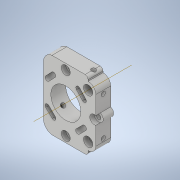
# Autodesk Inventor part: 20_Cube_Insert_Kinematic_VCAmount_Base_Thorlabs_Cage_smaller
Saved by Autodesk Inventor 2022.3 (Build 263350000, 350)
## iProperties
Created: 2019-07-01
Part Number: 20_Cube_Insert_Kinematic_VCAmount_Base_Thorlabs_Cage_smaller
Material: Generic
Document SubType Name: Modeling
Designer: diederichbenedict
Density: 1 g/cm^3
Appearance: Default
Author: diederichbenedict
Autodesk Inventor part; units mm, degrees
ref_plane "YZ Plane" through (0, 0, 0) normal (1, 0, 0) x (0, 1, 0)
ref_plane "Work Plane1" through (0, 0, 10) normal (0, 0, 1) x (1, 0, 0)
sketch "Sketch1" plane through (0, 0, 10) normal (0, 0, 1) x (1, 0, 0)
  line L0 (-4.0299, -0.3538) -> (-2.2322, 1.4439) construction
  arc A0 (-1.4439, 2.2322) -> (-2.2322, 1.4439) centre (-0.9299, 0.9299) ccw construction
  line L1 (-1.4439, 2.2322) -> (0.3538, 4.0299) construction
  line L2 (-37.8299, 42.8299) -> (-37.8299, 37.8299) construction
  line L3 (-37.8299, 37.8299) -> (-42.9208, 37.8299) construction
  line L4 (-37.8299, 42.2137) -> (-37.8299, 45.8299) construction
  line L5 (-37.8299, 45.8299) -> (-4.0299, 45.8299) construction
  line L6 (-4.0299, 45.8299) -> (-4.0299, 42.2137) construction
  line L7 (-4.0299, 4.0299) -> (0.3538, 4.0299) projected
  circle A1 centre (-20.9299, 20.9299) radius 17.5 projected
  line L8 (-20.9299, 58.9723) -> (17.1124, 20.9299) construction
  line L9 (17.1124, 20.9299) -> (-20.9299, -17.1124) construction
  line L10 (-20.9299, -17.1124) -> (-58.9723, 20.9299) construction
  line L11 (-58.9723, 20.9299) -> (-20.9299, 58.9723) construction
  line L12 (-20.9299, 58.9723) -> (-20.9299, -17.1124) construction
  line L13 (17.1124, 20.9299) -> (-58.9723, 20.9299) construction
  line L14 (-20.9299, 58.9723) -> (32.8701, 58.9723) construction
  line L15 (-43.4299, 43.4299) -> (1.5701, 43.4299) construction
  line L16 (1.5701, 43.4299) -> (1.5701, -1.5701) construction
  line L17 (1.5701, -1.5701) -> (-43.4299, -1.5701) construction
  line L18 (-43.4299, -1.5701) -> (-43.4299, 43.4299) construction
  line L19 (-43.4299, 43.4299) -> (1.5701, -1.5701) construction
  line L20 (1.5701, 43.4299) -> (-43.4299, -1.5701) construction
  line L21 (-43.4299, 5.3876) -> (-43.4299, 36.4723)
  line L22 (-43.4299, 36.4723) -> (-36.4723, 43.4299)
  line L23 (-36.4723, 43.4299) -> (-5.3876, 43.4299)
  line L24 (-5.3876, 43.4299) -> (1.5701, 36.4723)
  line L25 (1.5701, 36.4723) -> (1.5701, 5.3876)
  line L26 (1.5701, 5.3876) -> (-5.3876, -1.5701)
  line L27 (-5.3876, -1.5701) -> (-36.4723, -1.5701)
  line L28 (-36.4723, -1.5701) -> (-43.4299, 5.3876)
  line L29 (-4.0299, 42.2137) -> (-37.8299, 42.2137) projected
  line L30 (-4.0299, -0.3538) -> (-4.0299, 4.0299) projected
  point P0 (-37.8299, 4.0299)
  point P1 (-20.9299, 20.9299)
  dimension "d18" = 53.8
  dimension "d19" = 45
  dimension "d20" = 53.8
  dimension "d21" = 45
  dimension "d22" = 45
  constraints: 42 end point, 15 point on line, 5 midpoint, 4 parallel, 3 perpendicular, 2 horizontal, 1 equal length
  measures "d18" distance of L8.start L8.end
  measures "d19" angle of L8 L14
  measures "d20" distance of L8.end L9.end
  measures "d21" distance of L16.end L17.end
  measures "d22" distance of L15.end L16.end
extrude "Extrusion1" add sketch "Sketch1" along normal blind 10 contours L30 L26 L27 L28 L21 L22 L29 L24 L25 L7 | L7 L26 L30 | L29 L22 L23 L24 | A1
ref_plane "Work Plane2" through (-40.9959, 0.8639, 22.2359) normal (0, 0, 1) x (1, 0, 0)
sketch "Sketch3" plane through (0, 0, 10) normal (0, 0, -1) x (-1, 0, 0)
  line L0 (37.8299, -0.4701) -> (37.8299, 4.0299) construction
  line L1 (4.0299, 4.0299) -> (4.0299, -0.4701) construction
  line L2 (37.8299, -0.4701) -> (37.8299, 1.1886) construction
  line L3 (4.0299, -3.9701) -> (4.0299, -0.3538) construction
  line L4 (45.8299, 4.0299) -> (42.2137, 4.0299) construction
  line L5 (-0.3538, 4.0299) -> (-3.9701, 4.0299) construction
  line L6 (-3.9701, 37.8299) -> (-0.3538, 37.8299) construction
  line L7 (4.0299, 42.2137) -> (4.0299, 45.8299) construction
  line L8 (37.8299, 45.8299) -> (37.8299, 42.2137) construction
  line L9 (42.2137, 37.8299) -> (45.8299, 37.8299) construction
  line L10 (40.4657, 37.7299) -> (45.8299, 37.7299)
  line L11 (45.8299, 37.7299) -> (45.8299, 4.1299)
  line L12 (45.8299, 4.1299) -> (40.4657, 4.1299)
  line L13 (40.4657, 4.1299) -> (40.4657, 37.7299)
  line L14 (37.7299, 2.4952) -> (4.1299, 2.4952)
  line L15 (4.1299, 2.4952) -> (4.1299, -3.9701)
  line L16 (4.1299, -3.9701) -> (37.7299, -3.9701)
  line L17 (37.7299, -3.9701) -> (37.7299, 2.4952)
  line L18 (1.8946, 4.1299) -> (-3.9701, 4.1299)
  line L19 (-3.9701, 4.1299) -> (-3.9701, 37.7299)
  line L20 (-3.9701, 37.7299) -> (1.8946, 37.7299)
  line L21 (1.8946, 37.7299) -> (1.8946, 4.1299)
  line L22 (4.1299, 40.7326) -> (37.7299, 40.7326)
  line L23 (37.7299, 40.7326) -> (37.7299, 45.8299)
  line L24 (37.7299, 45.8299) -> (4.1299, 45.8299)
  line L25 (4.1299, 45.8299) -> (4.1299, 40.7326)
  point P0 (0, 0)
  dimension "d23" = 0.1
  dimension "d24" = 0.1
  dimension "d25" = 0.1
  dimension "d26" = 0.1
  dimension "d27" = 0.1
  constraints: 32 end point, 8 parallel, 4 horizontal, 4 perpendicular, 3 point on line
  measures "d23" distance between parallel lines of L8 L23
  measures "d24" distance between parallel lines of L7 L25
  measures "d25" distance between parallel lines of L6 L20
  measures "d26" distance between parallel lines of L5 L18
  measures "d27" distance between parallel lines of L1 L15
extrude "Extrusion3" add sketch "Sketch3" against normal up to surface (10 mm away)
sketch "Sketch4" plane through (0, 0, 20) normal (0, 0, 1) x (1, 0, 0)
  line L0 (3.9701, 4.1299) -> (0.3124, 4.1299) projected
  line L1 (3.9701, 37.7299) -> (3.9701, 4.1299) projected
  line L2 (0.3124, 37.7299) -> (3.9701, 37.7299) projected
  line L3 (0.3124, 37.7299) -> (-4.1299, 42.1723) projected
  line L4 (-4.1299, 45.8299) -> (-4.1299, 42.1723) projected
  line L5 (-37.7299, 45.8299) -> (-4.1299, 45.8299) projected
  line L6 (-37.7299, 42.1723) -> (-37.7299, 45.8299) projected
  line L7 (-37.7299, 42.1723) -> (-42.1723, 37.7299) projected
  line L8 (-45.8299, 37.7299) -> (-42.1723, 37.7299) projected
  line L9 (-45.8299, 4.1299) -> (-45.8299, 37.7299) projected
  line L10 (-42.1723, 4.1299) -> (-45.8299, 4.1299) projected
  line L11 (-42.1723, 4.1299) -> (-37.7299, -0.3124) projected
  line L12 (-37.7299, -3.9701) -> (-37.7299, -0.3124) projected
  line L13 (-4.1299, -3.9701) -> (-37.7299, -3.9701) projected
  line L14 (-4.1299, -0.3124) -> (-4.1299, -3.9701) projected
  line L15 (-4.1299, -0.3124) -> (0.3124, 4.1299) projected
  line L16 (-3.9799, 45.9799) -> (-3.9799, 42.2344)
  line L17 (-3.9799, 42.2344) -> (0.3745, 37.8799)
  line L18 (0.3745, 37.8799) -> (4.1201, 37.8799)
  line L19 (4.1201, 37.8799) -> (4.1201, 3.9799)
  line L20 (4.1201, 3.9799) -> (0.3745, 3.9799)
  line L21 (0.3745, 3.9799) -> (-3.9799, -0.3745)
  line L22 (-3.9799, -0.3745) -> (-3.9799, -4.1201)
  line L23 (-3.9799, -4.1201) -> (-37.8799, -4.1201)
  line L24 (-37.8799, -4.1201) -> (-37.8799, -0.3745)
  line L25 (-37.8799, -0.3745) -> (-42.2344, 3.9799)
  line L26 (-42.2344, 3.9799) -> (-45.9799, 3.9799)
  line L27 (-45.9799, 3.9799) -> (-45.9799, 37.8799)
  line L28 (-45.9799, 37.8799) -> (-42.2344, 37.8799)
  line L29 (-42.2344, 37.8799) -> (-37.8799, 42.2344)
  line L30 (-37.8799, 42.2344) -> (-37.8799, 45.9799)
  line L31 (-37.8799, 45.9799) -> (-3.9799, 45.9799)
  point P0 (0, 0)
  dimension "d34" = 0.15
  constraints: 32 end point, 15 other
  measures "d34" distance between parallel lines of L5 L31
extrude "Extrusion4" add sketch "Sketch4" against normal up to surface (10 mm away)
sketch "Sketch8" plane through (0, 0, 20) normal (0, 0, 1) x (1, 0, 0)
  circle A0 centre (-20.9299, 20.9299) radius 10
  line L0 (4.1201, 37.8799) -> (4.1201, 3.9799) projected
  line L1 (-37.8799, 45.9799) -> (-3.9799, 45.9799) projected
  point P0 (0, 0)
  point P1 (4.1201, 20.9299)
  point P2 (-20.9299, 45.9799)
  dimension "d61" = 20
  constraints: 2 midpoint, 1 centre point, 1 horizontal alignment, 1 vertical alignment
  measures "d61" diameter of A0
ref_plane "Work Plane3" through (-40.0572, 1.8027, 20) normal (-0.7071068, 0.7071068, 0) x (0.7071068, 0.7071068, 0)
sketch "Sketch5" plane through (0, 0, 20) normal (0, 0, 1) x (1, 0, 0)
  circle A0 centre (-20.9299, 20.9299) radius 29.7458 construction
  line L0 (4.1201, 37.8799) -> (4.1201, 3.9799) projected
  line L1 (-37.8799, 45.9799) -> (-3.9799, 45.9799) projected
  line L2 (-34.9299, 6.9299) -> (-6.9299, 6.9299) construction
  line L3 (-6.9299, 6.9299) -> (-6.9299, 34.9299) construction
  line L4 (-6.9299, 34.9299) -> (-34.9299, 34.9299) construction
  line L5 (-34.9299, 34.9299) -> (-34.9299, 6.9299) construction
  line L6 (-34.9299, 6.9299) -> (-6.9299, 34.9299) construction
  line L7 (-6.9299, 6.9299) -> (-34.9299, 34.9299) construction
  line L8 (-40.0218, 20.9299) -> (-20.9299, 40.0218)
  line L9 (-20.9299, 40.0218) -> (-1.838, 20.9299)
  line L10 (-1.838, 20.9299) -> (-20.9299, 1.838)
  line L11 (-20.9299, 1.838) -> (-40.0218, 20.9299)
  line L12 (-40.0218, 20.9299) -> (-1.838, 20.9299) construction
  line L13 (-20.9299, 40.0218) -> (-20.9299, 1.838) construction
  line L14 (-3.9799, -4.1201) -> (-37.8799, -4.1201) construction
  point P0 (0, 0)
  point P1 (4.1201, 20.9299)
  point P2 (-20.9299, 45.9799)
  point P3 (0, 0)
  point P4 (-20.9299, 20.9299)
  point P5 (-20.9299, 20.9299)
  point P6 (-20.9299, 45.9799)
  point P7 (-20.9299, -4.1201)
  point P8 (4.1201, 20.9299)
  dimension "d37" = 28
  dimension "d38" = 28
  dimension "d41" = 27
  dimension "d42" = 27
  constraints: 24 end point, 8 midpoint, 4 coincident, 4 parallel, 3 vertical alignment, 2 horizontal alignment, 2 perpendicular, 1 centre point, 1 horizontal
  measures "d37" distance of L4.end L3.end
  measures "d38" distance of L3.end L2.end
  measures "d41" distance of L10.end L8.start
  measures "d42" distance of L8.start L8.end
hole "Hole1" at (-20.9299, 40.0218, 20) at (-1.838, 20.9299, 20) at (-20.9299, 1.838, 20) at (-40.0218, 20.9299, 20) direction (0, 0, -1) diameter 2.955 end through all counterbore diameter 6 counterbore depth 3
sketch "Sketch6" plane through (0, 0, 20) normal (0, 0, 1) x (1, 0, 0)
  line L0 (-12.6431, 33.3435) -> (-8.598, 28.9122) construction
  line L1 (-13.7509, 32.3323) -> (-9.7058, 27.9009)
  line L2 (-7.4901, 29.9235) -> (-11.5353, 34.3548)
  arc A0 (-11.5353, 34.3548) -> (-13.6544, 34.4514) centre (-12.6431, 33.3435) ccw
  arc A1 (-9.7058, 27.9009) -> (-7.5867, 27.8044) centre (-8.598, 28.9122) ccw
  circle A2 centre (-20.9299, 40.0218) radius 3 construction
  line L3 (-3.9799, 45.9799) -> (-3.9799, 42.2344) projected
  line L4 (-37.8799, 45.9799) -> (-3.9799, 45.9799) projected
  line L5 (-37.8799, 42.2344) -> (-37.8799, 45.9799) projected
  line L6 (-42.2344, 37.8799) -> (-37.8799, 42.2344) projected
  line L7 (-45.9799, 37.8799) -> (-42.2344, 37.8799) projected
  line L8 (-45.9799, 3.9799) -> (-45.9799, 37.8799) projected
  line L9 (-42.2344, 3.9799) -> (-45.9799, 3.9799) projected
  line L10 (-37.8799, -0.3745) -> (-42.2344, 3.9799) projected
  line L11 (-37.8799, -4.1201) -> (-37.8799, -0.3745) projected
  line L12 (-3.9799, -4.1201) -> (-37.8799, -4.1201) projected
  line L13 (-3.9799, -0.3745) -> (-3.9799, -4.1201) projected
  line L14 (0.3745, 3.9799) -> (-3.9799, -0.3745) projected
  line L15 (4.1201, 3.9799) -> (0.3745, 3.9799) projected
  line L16 (4.1201, 37.8799) -> (4.1201, 3.9799) projected
  line L17 (0.3745, 37.8799) -> (4.1201, 37.8799) projected
  line L18 (-3.9799, 42.2344) -> (0.3745, 37.8799) projected
  circle A3 centre (-20.9299, 40.0218) radius 3 construction
  line L19 (-3.9799, 45.9799) -> (-3.9799, 42.2344) projected
  line L20 (-37.8799, 45.9799) -> (-3.9799, 45.9799) projected
  line L21 (-37.8799, 42.2344) -> (-37.8799, 45.9799) projected
  line L22 (-42.2344, 37.8799) -> (-37.8799, 42.2344) projected
  line L23 (-45.9799, 37.8799) -> (-42.2344, 37.8799) projected
  line L24 (-45.9799, 3.9799) -> (-45.9799, 37.8799) projected
  line L25 (-42.2344, 3.9799) -> (-45.9799, 3.9799) projected
  line L26 (-37.8799, -0.3745) -> (-42.2344, 3.9799) projected
  line L27 (-37.8799, -4.1201) -> (-37.8799, -0.3745) projected
  line L28 (-3.9799, -4.1201) -> (-37.8799, -4.1201) projected
  line L29 (-3.9799, -0.3745) -> (-3.9799, -4.1201) projected
  line L30 (0.3745, 3.9799) -> (-3.9799, -0.3745) projected
  line L31 (4.1201, 3.9799) -> (0.3745, 3.9799) projected
  line L32 (4.1201, 37.8799) -> (4.1201, 3.9799) projected
  line L33 (0.3745, 37.8799) -> (4.1201, 37.8799) projected
  line L34 (-3.9799, 42.2344) -> (0.3745, 37.8799) projected
  line L35 (-27.9727, 9.6345) -> (-32.2618, 13.8301)
  arc A4 (-30.0706, 7.4899) -> (-27.9494, 7.5133) centre (-29.0216, 8.5622) ccw
  arc A5 (-32.2618, 13.8301) -> (-34.383, 13.8068) centre (-33.3107, 12.7579) ccw
  line L36 (-34.3597, 11.6856) -> (-30.0706, 7.4899)
  line L37 (-33.3107, 12.7579) -> (-29.0216, 8.5622) construction
  arc A6 (-28.0504, 32.2739) -> (-28.0899, 34.3949) centre (-29.1306, 33.3146) ccw
  line L38 (-32.2131, 27.9529) -> (-28.0504, 32.2739)
  line L39 (-29.1306, 33.3146) -> (-32.2527, 30.0739) construction
  line L40 (-30.2109, 34.3553) -> (-34.3736, 30.0343)
  arc A7 (-34.3736, 30.0343) -> (-34.3341, 27.9133) centre (-33.2934, 28.9936) ccw
  line L41 (-45.9799, 3.9799) -> (-45.9799, 37.8799) projected
  line L42 (4.1201, 37.8799) -> (4.1201, 3.9799) projected
  circle A8 centre (-20.9299, 1.838) radius 3 projected
  circle A9 centre (-20.9299, 1.838) radius 1.4775 projected
  line L43 (-37.8799, 45.9799) -> (-3.9799, 45.9799) projected
  line L44 (-3.9799, -4.1201) -> (-37.8799, -4.1201) projected
  arc A10 (-28.0899, 34.3949) -> (-30.2109, 34.3553) centre (-29.1306, 33.3146) ccw
  arc A11 (-34.3341, 27.9133) -> (-32.2131, 27.9529) centre (-33.2934, 28.9936) ccw
  line L45 (-32.2527, 30.0739) -> (-33.2934, 28.9936) construction
  arc A12 (-34.383, 13.8068) -> (-34.3597, 11.6856) centre (-33.3107, 12.7579) ccw
  arc A13 (-27.9494, 7.5133) -> (-27.9727, 9.6345) centre (-29.0216, 8.5622) ccw
  arc A14 (-13.6544, 34.4514) -> (-13.7509, 32.3323) centre (-12.6431, 33.3435) ccw
  arc A15 (-7.5867, 27.8044) -> (-7.4901, 29.9235) centre (-8.598, 28.9122) ccw
  arc A16 (-7.4948, 11.7377) -> (-7.4948, 13.859) centre (-8.5554, 12.7983) ccw
  line L46 (-11.7374, 7.495) -> (-7.4948, 11.7377)
  line L47 (-12.7981, 8.5557) -> (-9.6161, 11.7377) construction
  line L48 (-9.6161, 13.859) -> (-13.8587, 9.6164)
  arc A17 (-13.8587, 9.6164) -> (-13.8587, 7.4951) centre (-12.7981, 8.5557) ccw
  arc A18 (-13.8587, 7.4951) -> (-11.7374, 7.495) centre (-12.7981, 8.5557) ccw
  arc A19 (-7.4948, 13.859) -> (-9.6161, 13.859) centre (-8.5554, 12.7983) ccw
  line L49 (-9.6161, 11.7377) -> (-8.5554, 12.7983) construction
  circle A20 centre (-20.9299, 1.838) radius 3 projected
  circle A21 centre (-20.9299, 40.0218) radius 3 construction
  circle A22 centre (-1.838, 20.9299) radius 3 construction
  circle A23 centre (-40.0218, 20.9299) radius 3 projected
  line L50 (-3.9799, 45.9799) -> (-3.9799, 42.2344) projected
  line L51 (-37.8799, 45.9799) -> (-3.9799, 45.9799) projected
  line L52 (-37.8799, 42.2344) -> (-37.8799, 45.9799) projected
  line L53 (-42.2344, 37.8799) -> (-37.8799, 42.2344) projected
  line L54 (-45.9799, 37.8799) -> (-42.2344, 37.8799) projected
  line L55 (-45.9799, 3.9799) -> (-45.9799, 37.8799) projected
  line L56 (-42.2344, 3.9799) -> (-45.9799, 3.9799) projected
  line L57 (-37.8799, -0.3745) -> (-42.2344, 3.9799) projected
  line L58 (-37.8799, -4.1201) -> (-37.8799, -0.3745) projected
  line L59 (-3.9799, -4.1201) -> (-37.8799, -4.1201) projected
  line L60 (-3.9799, -0.3745) -> (-3.9799, -4.1201) projected
  line L61 (0.3745, 3.9799) -> (-3.9799, -0.3745) projected
  line L62 (4.1201, 3.9799) -> (0.3745, 3.9799) projected
  line L63 (4.1201, 37.8799) -> (4.1201, 3.9799) projected
  line L64 (0.3745, 37.8799) -> (4.1201, 37.8799) projected
  line L65 (-3.9799, 42.2344) -> (0.3745, 37.8799) projected
  circle A24 centre (-20.9299, 1.838) radius 3 projected
  circle A25 centre (-20.9299, 40.0218) radius 3 projected
  circle A26 centre (-1.838, 20.9299) radius 3 projected
  circle A27 centre (-40.0218, 20.9299) radius 3 projected
  line L66 (-3.9799, 45.9799) -> (-3.9799, 42.2344) projected
  line L67 (-37.8799, 45.9799) -> (-3.9799, 45.9799) projected
  line L68 (-37.8799, 42.2344) -> (-37.8799, 45.9799) projected
  line L69 (-42.2344, 37.8799) -> (-37.8799, 42.2344) projected
  line L70 (-45.9799, 37.8799) -> (-42.2344, 37.8799) projected
  line L71 (-45.9799, 3.9799) -> (-45.9799, 37.8799) projected
  line L72 (-42.2344, 3.9799) -> (-45.9799, 3.9799) projected
  line L73 (-37.8799, -0.3745) -> (-42.2344, 3.9799) projected
  line L74 (-37.8799, -4.1201) -> (-37.8799, -0.3745) projected
  line L75 (-3.9799, -4.1201) -> (-37.8799, -4.1201) projected
  line L76 (-3.9799, -0.3745) -> (-3.9799, -4.1201) projected
  line L77 (0.3745, 3.9799) -> (-3.9799, -0.3745) projected
  line L78 (4.1201, 3.9799) -> (0.3745, 3.9799) projected
  line L79 (4.1201, 37.8799) -> (4.1201, 3.9799) projected
  line L80 (0.3745, 37.8799) -> (4.1201, 37.8799) projected
  line L81 (-3.9799, 42.2344) -> (0.3745, 37.8799) projected
  circle A28 centre (-20.9299, 20.9299) radius 16 construction
  circle A29 centre (-20.9299, 1.838) radius 3 projected
  circle A30 centre (-20.9299, 40.0218) radius 3 projected
  circle A31 centre (-1.838, 20.9299) radius 3 projected
  circle A32 centre (-40.0218, 20.9299) radius 3 projected
  line L82 (-3.9799, 45.9799) -> (-3.9799, 42.2344) projected
  line L83 (-37.8799, 45.9799) -> (-3.9799, 45.9799) projected
  line L84 (-37.8799, 42.2344) -> (-37.8799, 45.9799) projected
  line L85 (-42.2344, 37.8799) -> (-37.8799, 42.2344) projected
  line L86 (-45.9799, 37.8799) -> (-42.2344, 37.8799) projected
  line L87 (-45.9799, 3.9799) -> (-45.9799, 37.8799) projected
  line L88 (-42.2344, 3.9799) -> (-45.9799, 3.9799) projected
  line L89 (-37.8799, -0.3745) -> (-42.2344, 3.9799) projected
  line L90 (-37.8799, -4.1201) -> (-37.8799, -0.3745) projected
  line L91 (-3.9799, -4.1201) -> (-37.8799, -4.1201) projected
  line L92 (-3.9799, -0.3745) -> (-3.9799, -4.1201) projected
  line L93 (0.3745, 3.9799) -> (-3.9799, -0.3745) projected
  line L94 (4.1201, 3.9799) -> (0.3745, 3.9799) projected
  line L95 (4.1201, 37.8799) -> (4.1201, 3.9799) projected
  line L96 (0.3745, 37.8799) -> (4.1201, 37.8799) projected
  line L97 (-3.9799, 42.2344) -> (0.3745, 37.8799) projected
  circle A33 centre (-1.838, 20.9299) radius 3 projected
  circle A34 centre (-20.9299, 40.0218) radius 3 projected
  line L98 (-3.9799, 45.9799) -> (-3.9799, 42.2344) projected
  point P0 (-10.6205, 31.1279)
  point P1 (-45.9799, 20.9299)
  point P2 (-40.7289, 40.7289)
  point P3 (-31.1662, 10.66)
  point P4 (66.7709, 47.2309)
  point P5 (-45.9801, 20.9299)
  point P6 (-11.7284, 30.1166)
  point P7 (-30.1579, 30.1577)
  point P8 (-40.0572, 40.0572)
  point P9 (-32.2151, 9.5878)
  point P10 (-32.2923, 32.1948)
  point P11 (-45.9801, 20.9299)
  point P12 (-40.0573, 1.8027)
  point P13 (-40.0573, 1.8027)
  point P14 (-10.6767, 10.677)
  point P15 (-9.6161, 9.6164)
  point P16 (-9.5127, 32.1392)
  point P17 (4.1201, 20.9299)
  point P18 (-20.9299, -4.1201)
  point P19 (-20.9299, 45.9799)
  dimension "d52" = 3
  dimension "d53" = 3
  dimension "d87" = 3
  dimension "d88" = 3
  dimension "d92" = 3
  dimension "d159" = 3
  dimension "d160" = 3
  dimension "d178" = 9
  dimension "d179" = 9
  dimension "d180" = 9
  dimension "d181" = 9
  dimension "d183" = 32
  constraints: 38 point on circle, 34 end point, 32 tangent, 17 centre point, 12 midpoint, 10 point on line, 4 parallel, 3 vertical alignment, 2 horizontal alignment, 1 coincident, 1 other
  measures "d52" distance of point (-10.621, 31.128) L0.end
  measures "d53" diameter of A1
  measures "d87" distance of point (-31.166, 10.66) L37.end
  measures "d88" diameter of A4
  measures "d92" diameter of A7
  measures "d159" distance of point (-10.677, 10.677) L49.end
  measures "d160" diameter of A16
  measures "d178" distance of A1.end A0.end
  measures "d179" distance of A7.end A6.end
  measures "d180" distance of A4.end A5.end
  measures "d181" distance of A18.start A16.end
  measures "d183" diameter of A28
extrude "Extrusion5" cut sketch "Sketch6" against normal through all contours A14 A0 L2 A15 A1 L1 | A13 A4 L36 A12 A5 L35 | L38 A11 A7 L40 A10 A6 | L46 A18 A17 L48 A19 A16
extrude "Extrusion6" cut sketch "Sketch8" against normal through all
sketch "Sketch2" plane through (0, 0, 20) normal (0, 0, 1) x (1, 0, 0)
  circle A0 centre (-35.9299, 35.9299) radius 3.0099 construction
  circle A1 centre (-5.93, 35.9299) radius 3.0099 construction
  circle A2 centre (-5.93, 5.93) radius 3.0099 construction
  circle A3 centre (-35.9299, 5.93) radius 3.0099 construction
  circle A4 centre (-35.9299, 35.9299) radius 3.125 construction
  circle A5 centre (-5.93, 35.9299) radius 3.125 construction
  circle A6 centre (-5.93, 5.93) radius 3.125 construction
  circle A7 centre (-35.9299, 5.93) radius 3.125 construction
  line L0 (1.5701, 5.3876) -> (1.5701, 36.4723) projected
  line L1 (-5.3876, 43.4299) -> (-36.4723, 43.4299) projected
  line L2 (-36.4723, 43.4299) -> (-43.4299, 36.4723) projected
  line L3 (-34.3736, 30.0343) -> (-30.2109, 34.3553) projected
  line L4 (-9.7058, 27.9009) -> (-13.7509, 32.3323) projected
  line L5 (-30.0706, 7.4899) -> (-34.3597, 11.6856) projected
  circle A8 centre (-5.93, 5.93) radius 5.1
  circle A9 centre (-5.93, 35.9299) radius 5.1
  point P0 (0, 0)
  point P1 (-20.9299, 20.9299)
  point P2 (1.5701, 20.9299)
  point P3 (-20.9299, 43.4299)
  point P4 (-35.9299, 35.9299)
  point P5 (-38.1396, 38.1396)
  point P6 (-36.7387, 32.9114)
  point P7 (-32.9114, 36.7387)
  point P8 (-26.8708, 10.3349)
  point P9 (-4.0799, 33.1904)
  point P10 (-4.1189, 8.6799)
  point P11 (-9.902, 8.6799)
  dimension "d31" = 6.25
  dimension "d32" = 6.25
  dimension "d33" = 6.25
  dimension "d102" = 6.25
  dimension "d110" = 19.0707
  dimension "d140" = 10.2
  dimension "d141" = 10.2
  constraints: 6 centre point, 3 point on circle, 2 midpoint, 1 coincident, 1 horizontal alignment, 1 vertical alignment
  measures "d31" diameter of A5
  measures "d32" diameter of A6
  measures "d33" diameter of A7
  measures "d102" diameter of A4
  measures "d110" distance from line of L3 point (-26.871, 10.335)
  measures "d140" diameter of A8
  measures "d141" diameter of A9
sketch "Sketch9" plane through (4.1201, 3.9799, 20) normal (1, 0, 0) x (0, 0, -1)
  line L0 (0, 0) -> (10, 0) projected
  line L1 (0, 33.9) -> (10, 33.9) projected
  point P0 (20, -3.9799)
  point P1 (5, 4)
  point P2 (5, 0)
  point P3 (5, 29.9)
  point P4 (5, 33.9)
  dimension "d64" = 4
  dimension "d65" = 4
  constraints: 2 midpoint, 2 vertical alignment
  measures "d64" distance from line of L0 point (5, 4)
  measures "d65" distance from line of L1 point (5, 29.9)
hole "Hole2" at (4.1201, 7.9799, 15) at (4.1201, 33.8799, 15) direction (-1, 0, 0) diameter 2.9 depth 10 tip angle 118
extrude "Extrusion7" [suppressed]
sketch "Sketch10" plane through (0, 0, 20) normal (0, 0, 1) x (1, 0, 0)
  line L0 (-37.8799, 45.9799) -> (-3.9799, 45.9799) projected
  line L1 (-36.4799, 45.9799) -> (-37.0382, 45.9799)
  line L2 (-42.2344, 3.9799) -> (-45.9799, 3.9799) projected
  line L3 (-45.9799, 3.9799) -> (-42.2344, 3.9799)
  line L4 (-3.9799, 45.9799) -> (-3.9799, 42.2344) projected
  line L5 (-3.9799, 43.9799) -> (-5.9799, 43.9799)
  line L6 (-36.4799, 45.9799) -> (-34.3858, 45.9799)
  line L7 (-3.9799, 43.9799) -> (-3.9799, 45.9799)
  line L8 (-3.9799, -4.1201) -> (-3.9799, -2.1201)
  line L9 (-3.9799, -0.3745) -> (-3.9799, -4.1201) projected
  line L10 (-3.9799, -2.1201) -> (-5.7255, -2.1201)
  line L11 (-34.3858, 45.9799) -> (-28.9151, 45.9799)
  circle A0 centre (-5.93, 5.93) radius 3.0099 projected
  circle A1 centre (-5.93, 35.9299) radius 3.0099 projected
  arc A2 (-0.83, 5.93) -> (-5.9799, 0.8302) centre (-5.93, 5.93) ccw
  arc A3 (-3.9799, 40.6424) -> (-5.9799, 41.0297) centre (-5.93, 35.9299) ccw
  line L12 (-3.9799, 43.9799) -> (-3.9799, 40.6424)
  line L13 (-0.83, 35.9299) -> (-0.83, 23.7555)
  line L14 (-3.9799, -0.3745) -> (-3.9799, 1.2175)
  line L15 (-5.9799, -2.1201) -> (-5.9799, 0.8302)
  line L16 (-5.9799, 41.0297) -> (-5.9799, 43.9799)
  circle A4 centre (-1.838, 20.9299) radius 3 projected
  circle A5 centre (-1.838, 20.9299) radius 1.4775 projected
  circle A6 centre (-1.838, 20.9299) radius 3 projected
  line L17 (-3.9799, -4.1201) -> (-0.83, -4.1201)
  line L18 (6.2025, -4.1201) -> (6.2025, 45.9799)
  line L19 (6.2025, 45.9799) -> (4.1201, 45.9799)
  circle A7 centre (-5.93, 5.93) radius 3.1099
  circle A8 centre (-5.93, 35.9299) radius 3.1099
  arc A9 (-3.9799, 1.2175) -> (-1.2175, 3.9799) centre (-5.93, 5.93) ccw
  arc A10 (-1.2175, 3.9799) -> (-0.83, 5.93) centre (-5.93, 5.93) ccw
  line L20 (-0.83, 18.1044) -> (-0.83, 5.93)
  line L21 (-0.83, 23.7555) -> (-0.83, 18.1044)
  arc A11 (-0.83, 35.9299) -> (-1.2175, 37.8799) centre (-5.93, 35.9299) ccw
  arc A12 (-5.9799, 41.0297) -> (-10.6424, 37.8799) centre (-5.93, 35.9299) ccw
  line L22 (0.3745, 3.9799) -> (-3.9799, -0.3745) projected
  line L23 (-3.9799, -0.3745) -> (-3.9799, -2.1201)
  line L24 (-3.9799, 1.2175) -> (-3.9799, -0.3745)
  line L25 (-5.9799, 41.0297) -> (-5.9799, 43.9799)
  line L26 (-3.9799, 43.9799) -> (-3.9799, 40.6424)
  line L27 (-3.9799, -0.3745) -> (-3.9799, -2.1201)
  arc A13 (-5.9799, 0.8302) -> (-3.9799, 1.2175) centre (-5.93, 5.93) ccw
  line L28 (-5.7255, -2.1201) -> (-5.9799, -2.1201)
  arc A14 (-10.6424, 37.8799) -> (-0.83, 35.9299) centre (-5.93, 35.9299) ccw
  arc A15 (-1.2175, 37.8799) -> (-3.9799, 40.6424) centre (-5.93, 35.9299) ccw
  line L29 (-0.83, 45.9799) -> (-3.9799, 45.9799)
  line L30 (-5.9799, 45.9799) -> (-3.9799, 45.9799)
  line L31 (-28.9151, 45.9799) -> (-5.9799, 45.9799)
  line L32 (-37.0382, 45.9799) -> (-37.8799, 45.9799)
  line L33 (-5.9799, -4.1201) -> (-3.9799, -4.1201)
  line L34 (4.1201, 37.8799) -> (4.1201, 3.9799) projected
  line L35 (-3.9799, -4.1201) -> (-37.8799, -4.1201) projected
  line L36 (-5.9799, -4.1201) -> (-7.7255, -4.1201)
  line L37 (-37.8799, -0.3745) -> (-42.2344, 3.9799) projected
  line L38 (-37.8799, -4.1201) -> (-37.8799, -2.1201)
  line L39 (-37.8799, -0.3745) -> (-42.2344, 3.9799)
  line L40 (-42.2344, 3.9799) -> (-45.9799, 3.9799)
  line L41 (-45.9799, 3.9799) -> (-45.9799, 37.8799) projected
  line L42 (-45.9799, 3.9799) -> (-45.9799, 7.7255)
  line L43 (-42.2344, 37.8799) -> (-37.8799, 42.2344) projected
  line L44 (-45.9799, 37.8799) -> (-42.2344, 37.8799)
  line L45 (-42.2344, 37.8799) -> (-37.8799, 42.2344)
  line L46 (-37.8799, 45.9799) -> (-3.9799, 45.9799) projected
  line L47 (-37.8799, 42.2344) -> (-37.8799, 43.9799)
  line L48 (-37.8799, 43.9799) -> (-37.8799, 45.9799)
  line L49 (-45.9799, 34.1344) -> (-45.9799, 37.8799)
  line L50 (-45.9799, 7.7255) -> (-45.9799, 34.1344)
  line L51 (-37.8799, -2.1201) -> (-37.8799, -0.3745)
  line L52 (-34.1344, -4.1201) -> (-37.8799, -4.1201)
  line L53 (-7.7255, -4.1201) -> (-25.1869, -4.1201)
  line L54 (-0.83, -4.1201) -> (6.2025, -4.1201)
  line L55 (4.1201, 45.9799) -> (-0.83, 45.9799)
  line L56 (-5.9799, 43.9799) -> (-20.9387, 43.9799)
  line L57 (-5.9799, -2.1201) -> (-20.2466, -2.1201)
  line L58 (-25.1869, -4.1201) -> (-34.1344, -4.1201)
  line L59 (-30.0706, 7.4899) -> (-34.3597, 11.6856) projected
  line L60 (-34.3736, 30.0343) -> (-30.2109, 34.3553) projected
  arc A16 (-34.3736, 30.0343) -> (-32.2131, 27.9529) centre (-33.2934, 28.9936) ccw projected
  line L61 (-20.9387, 43.9799) -> (-28.4882, 43.9799)
  line L62 (-20.2466, -2.1201) -> (-24.8391, -2.1201)
  line L63 (-35.8495, 37.5372) -> (-35.8495, 28.5023)
  line L64 (4.1201, 3.9799) -> (0.3745, 3.9799) projected
  arc A17 (-30.2109, 43.9799) -> (-35.8405, 37.8799) centre (-29.3495, 37.5372) ccw
  arc A18 (-35.8405, 37.8799) -> (-35.8495, 37.5372) centre (-29.3495, 37.5372) ccw
  line L65 (-35.8495, 28.5023) -> (-35.8495, 4.1595)
  line L66 (-24.8391, -2.1201) -> (-30.2109, -2.1201)
  line L67 (-28.4882, 43.9799) -> (-30.2109, 43.9799)
  arc A19 (-35.8495, 4.1595) -> (-30.2109, -2.1201) centre (-29.3516, 4.3229) ccw
  point P0 (0, 0)
  point P1 (-0.83, 24.166)
  point P2 (-0.83, 23.7555)
  point P3 (1.162, 20.9299)
  point P4 (1.162, 20.9299)
  dimension "d127" = 2
  dimension "d137" = 10.2
  dimension "d138" = 10.2
  dimension "d139" = 2
  dimension "d142" = 0.1
  dimension "d143" = 0.1
  dimension "d147" = 6.0198
  dimension "d202" = 2
  dimension "d206" = 6.5
  dimension "d207" = 6.5
  constraints: 109 end point, 27 point on circle, 23 point on line, 17 perpendicular, 14 centre point, 14 collinear, 14 horizontal, 12 parallel, 10 tangent, 4 vertical, 1 coincident
  measures "d127" distance between parallel lines of L0 L5
  measures "d137" diameter of A2
  measures "d138" diameter of A3
  measures "d139" distance between parallel lines of L15 L9
  measures "d142" radial gap between concentric circles of A0 A7
  measures "d143" radial gap between concentric circles of A1 A8
  measures "d147" diameter of A1
  measures "d202" distance between parallel lines of L53 L57
  measures "d206" radius of A17
  measures "d207" radius of A19
extrude "Extrusion8" cut sketch "Sketch10" against normal through all contours L0 L4 L5 L56 L61 L67 A17 A18 L63 L65 A19 L66 L62 L57 L28 L10 L8 L33 L35 L38 L51 L37 L2 L41 L44 L43 L47 L48 | L29 L55 L19 L18 L54 L17 L8 L9 L14 A9 A10 L20 A4 L13 A11 A15 L12 L4 | L4 L12 A3 L16 L5 | L10 L28 L15 A13 L14 L9 | A0 | A1 | A7 | A8
fillet "Fillet1" radius 2 2 edges at (-5.9799, 43.9799, 15) (-5.9799, -2.1201, 15)
sketch "Sketch11" plane through (-33.5228, 43.9799, 20) normal (0, 1, 0) x (1, 0, 0)
  line L0 (25.5429, 10) -> (25.5429, 0) projected
  circle A0 centre (25.5429, 5.6058) radius 1.45
  line L1 (20.126, 0) -> (20.126, 10) projected
  line L2 (-0.749, 0) -> (20.126, 0) projected
  line L3 (-0.749, 0) -> (-0.749, 10) projected
  line L4 (20.126, 10) -> (-0.749, 10) projected
  point P0 (33.5228, 20)
  dimension "d166" = 2.9
  constraints: 1 centre point, 1 point on line
  measures "d166" diameter of A0
extrude "Extrusion9" cut sketch "Sketch11" against normal blind 9 contours A0 L0 | L0 A0
sketch "Sketch13" plane through (-7.4901, 29.9235, 10) normal (-0.7385575, -0.6741905, 0) x (0, 0, 1)
  circle A0 centre (5, 3.1694) radius 1.45
  line L0 (10, 6.4941) -> (10, 0.2743) projected
  line L1 (10, 3.1694) -> (0, 3.1694) construction
  line L2 (0, 0.2743) -> (0, 6.4941) projected
  line L3 (7, -9.0456) -> (10, -9.0456) projected
  point P0 (-10, -27.15)
  dimension "d184" = 12.215
  dimension "d185" = 2.9
  constraints: 2 end point, 2 point on line, 1 centre point, 1 coincident, 1 horizontal, 1 midpoint
  measures "d184" distance from line of L3 A0.centre
  measures "d185" diameter of A0
extrude "Extrusion11" cut sketch "Sketch13" along normal blind 10
pattern_circular "Circular Pattern5" count 4 over 360 about axis through (-20.9299, 20.9299, 20) along (0, 0, -1) of "Extrusion11"
sketch "Sketch14" plane through (-34.7418, -2.1201, 10) normal (0, -1, 0) x (1, 0, 0)
  line L0 (26.7619, 10) -> (26.7619, 0) projected
  circle A0 centre (26.7619, 5) radius 1.45
  line L1 (28.7619, 0) -> (28.7619, 10) projected
  point P0 (34.7418, -10)
  point P1 (28.7619, 5)
  dimension "d194" = 2.9
  constraints: 3 midpoint, 1 centre point, 1 coincident
  measures "d194" diameter of A0
extrude "Extrusion12" cut sketch "Sketch14" against normal blind 9
equation "\"d42\" = d41"
equation "\"d65\" = d64"
body "Solid1"
